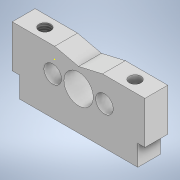
# Autodesk Inventor part: rod holder on
Saved by Autodesk Inventor 2022 (Build 260153000, 153)
## iProperties
Created: 2022-04-17
Part Number: rod holder on
Material: Generic
Document SubType Name: Modeling
Designer: vitalii
Density: 1 g/cm^3
Appearance: Default
Author: vitalii
Autodesk Inventor part; units mm, degrees
ref_plane "YZ Plane" through (0, 0, 0) normal (1, 0, 0) x (0, 1, 0)
ref_plane "XZ Plane" through (0, 0, 0) normal (0, 1, 0) x (-1, 0, 0)
ref_plane "XY Plane" through (0, 0, 0) normal (0, 0, 1) x (1, 0, 0)
sketch "Sketch1" plane through (0, 0, 0) normal (0, 0, 1) x (1, 0, 0)
  point P0 (0, 0)
sketch "Sketch2" plane through (0, 0, 0) normal (0, 0, 1) x (1, 0, 0)
  line L0 (-22.9271, 6.1236) -> (-22.9271, -16.8764)
  line L1 (-22.9271, -16.8764) -> (48.9029, -16.8764)
  line L2 (48.9029, -16.8764) -> (48.9029, 6.1236)
  line L3 (48.9029, 6.1236) -> (-22.9271, 6.1236)
  point P0 (0, 0)
  dimension "d0" = 23
  dimension "d1" = 71.83
  constraints: 8 end point, 2 perpendicular, 1 horizontal, 1 vertical
  measures "d0" distance of L0.start L0.end
  measures "d1" distance of L0.end L1.end
extrude "Extrusion1" add sketch "Sketch2" against normal blind 12.36
sketch "Sketch3" plane through (0, 0, 0) normal (0, 0, 1) x (1, 0, 0)
  point P0 (0, 0)
sketch "Sketch4" plane through (0, 0, 0) normal (0, 0, 1) x (1, 0, 0)
  line L0 (0.0479, 6.1236) -> (25.9279, 6.1236)
  line L1 (25.9279, 6.1236) -> (12.9879, 3.1378)
  line L2 (12.9879, 3.1378) -> (0.0479, 6.1236)
  line L3 (48.9029, 6.1236) -> (-22.9271, 6.1236) projected
  line L4 (48.9029, -16.8764) -> (48.9029, 6.1236) projected
  circle A0 centre (12.9879, -7.3764) radius 7.9375
  circle A1 centre (-1.0121, -7.3764) radius 4.7625
  circle A2 centre (26.9879, -7.3764) radius 4.7625
  line L5 (-22.9271, -16.8764) -> (48.9029, -16.8764) projected
  line L6 (-19.0821, -16.8764) -> (45.0579, -16.8764)
  line L7 (45.0579, -16.8764) -> (45.0579, -28.1264)
  line L8 (45.0579, -28.1264) -> (-19.0821, -28.1264)
  line L9 (-19.0821, -28.1264) -> (-19.0821, -16.8764)
  line L10 (-22.9271, 6.1236) -> (-22.9271, -16.8764) projected
  point P0 (0, 0)
  dimension "d4" = 25.88
  dimension "d7" = 13.28
  dimension "d8" = 0
  dimension "d10" = 2.9858
  dimension "d11" = 35.915
  dimension "d12" = 15.875
  dimension "d13" = 9.5
  dimension "d14" = 14
  dimension "d15" = 9.5
  dimension "d16" = 9.5
  dimension "d17" = 14
  dimension "d18" = 9.525
  dimension "d19" = 9.525
  dimension "d20" = 64.14
  dimension "d21" = 11.25
  dimension "d22" = 3.845
  dimension "d23" = 0
  constraints: 14 end point, 3 centre point, 3 perpendicular, 1 collinear, 1 horizontal
  measures "d4" distance of L0.start L0.end
  measures "d7" distance of L0.end L1.end
  measures "d8" distance between parallel lines of L3 L0
  measures "d10" vertical distance of L1.end L0.start
  measures "d11" distance from line of L4 L1.end
  measures "d12" diameter of A0
  measures "d13" distance from line of L5 A0.centre
  measures "d14" distance of A1.centre A0.centre
  measures "d15" distance from line of L5 A1.centre
  measures "d16" distance from line of L5 A2.centre
  measures "d17" distance of A0.centre A2.centre
  measures "d18" diameter of A1
  measures "d19" diameter of A2
  measures "d20" distance of L6.start L6.end
  measures "d21" distance of L6.end L7.end
  measures "d22" distance between parallel lines of L10 L9
  measures "d23" distance between parallel lines of L5 L6
extrude "Extrusion2" cut sketch "Sketch4" against normal blind 12.36 contours L0 L1 L2 | A0 | A1 | A2
extrude "Extrusion3" add sketch "Sketch4" against normal blind 12.36 contours L5 L7 L8 L9
sketch "Sketch5" plane through (-22.9271, 6.1236, 0) normal (0, 1, 0) x (1, 0, 0)
  circle A0 centre (11.4875, 6.18) radius 3.175
  line L0 (0, 12.36) -> (22.975, 12.36) projected
  line L1 (0, 0) -> (0, 12.36) projected
  circle A1 centre (60.342, 6.18) radius 3.175
  line L2 (71.83, 0) -> (71.83, 12.36) projected
  point P0 (22.9271, 0)
  dimension "d28" = 6.18
  dimension "d29" = 6.35
  dimension "d30" = 11.4875
  dimension "d31" = 6.35
  dimension "d32" = 11.488
  constraints: 2 centre point
  measures "d28" distance from line of A0.centre L0
  measures "d29" diameter of A0
  measures "d30" distance from line of L1 A0.centre
  measures "d31" diameter of A1
  measures "d32" distance from line of L2 A1.centre
extrude "Extrusion4" cut sketch "Sketch5" against normal blind 13
thread "Thread1" size "1/4-20 UNC" class "2B" standard "ANSI Unified Screw Threads" full length
body "Solid1"
